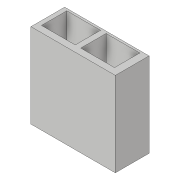
# Autodesk Inventor part: exploration1.1
Saved by Autodesk Inventor 2019 (Build 230136000, 136)
## iProperties
Created: 2020-02-18
Part Number: exploration1.1
Material: Generic
Document SubType Name: Modeling
Designer: Sandeep Shankar P
Density: 1 g/cm^3
Appearance: Default
Author: Sandeep Shankar P
Autodesk Inventor part; units mm, degrees
ref_plane "YZ Plane" through (0, 0, 0) normal (1, 0, 0) x (0, 1, 0)
ref_plane "XZ Plane" through (0, 0, 0) normal (0, 1, 0) x (-1, 0, 0)
ref_plane "XY Plane" through (0, 0, 0) normal (0, 0, 1) x (1, 0, 0)
sketch "Sketch1" plane through (0, 0, 0) normal (0, 0, 1) x (1, 0, 0)
  line L0 (-100, -49.8579) -> (100, -49.8579)
  line L1 (100, -49.8579) -> (100, 150.1421)
  line L2 (100, 150.1421) -> (-100, 150.1421)
  line L3 (-100, 150.1421) -> (-100, -49.8579)
  line L4 (-100, -49.8579) -> (100, 150.1421) construction
  line L5 (100, -49.8579) -> (-100, 150.1421) construction
  point P0 (0, 50.1421)
  dimension "d13" = 200
  dimension "d14" = 200
  dimension "d17" = 200
  constraints: 12 end point, 2 midpoint, 2 parallel, 1 horizontal, 1 perpendicular
  measures "d13" distance between parallel lines of L1 L3
  measures "d14" distance between parallel lines of L2 L0
  measures "d17" distance of L0.start L0.end
extrude "Extrusion1" add sketch "Sketch1" along normal blind 80
sketch "Sketch2" plane through (-100, 150.1421, 0) normal (0, 1, 0) x (1, 0, 0)
  line L0 (90, -65) -> (10, -65)
  line L1 (10, -65) -> (10, -5)
  line L2 (10, -5) -> (90, -5)
  line L3 (90, -5) -> (90, -65)
  line L4 (90, -65) -> (10, -5) construction
  line L5 (10, -65) -> (90, -5) construction
  line L6 (0, 0) -> (0, -80) projected
  line L7 (200, 0) -> (0, 0) projected
  point P0 (100, 0)
  point P1 (50, -35)
  dimension "d7" = 80
  dimension "d8" = 60
  dimension "d9" = 10
  dimension "d10" = 5
  constraints: 12 end point, 2 midpoint, 2 parallel, 1 horizontal, 1 perpendicular
  measures "d7" distance of L1.end L2.end
  measures "d8" distance of L0.end L1.end
  measures "d9" distance between parallel lines of L6 L1
  measures "d10" distance between parallel lines of L7 L2
extrude "Extrusion2" cut sketch "Sketch2" against normal blind 80
sketch "Sketch3" plane through (0, 0, 0) normal (0, 0, -1) x (-1, 0, 0)
  circle A0 centre (-10, 30.1421) radius 25
  line L0 (100, -49.8579) -> (-100, -49.8579) projected
  line L1 (-100, -49.8579) -> (-100, 150.1421) projected
  point P0 (0, 0)
  dimension "d19" = 50
  dimension "d20" = 80
  dimension "d21" = 90
  constraints: 1 centre point
  measures "d19" diameter of A0
  measures "d20" distance from line of L0 A0.centre
  measures "d21" distance from line of L1 A0.centre
extrude "Extrusion3" cut sketch "Sketch3" against normal blind 70
sketch "Sketch4" plane through (-100, 150.1421, 0) normal (0, 1, 0) x (1, 0, 0)
  line L0 (183.0719, -5) -> (103.0719, -5)
  line L1 (103.0719, -5) -> (103.0719, -65)
  line L2 (103.0719, -65) -> (183.0719, -65)
  line L3 (183.0719, -65) -> (183.0719, -5)
  line L4 (183.0719, -5) -> (103.0719, -65) construction
  line L5 (103.0719, -5) -> (183.0719, -65) construction
  line L6 (200, 0) -> (0, 0) projected
  point P0 (100, 0)
  point P1 (143.0719, -35)
  dimension "d24" = 80
  dimension "d25" = 60
  dimension "d26" = 5
  constraints: 12 end point, 2 midpoint, 2 parallel, 1 horizontal, 1 perpendicular
  measures "d24" distance of L2.end L1.end
  measures "d25" distance between parallel lines of L2 L0
  measures "d26" distance between parallel lines of L0 L6
extrude "Extrusion4" cut sketch "Sketch4" against normal blind 80
sketch "Sketch5" plane through (0, 0, 0) normal (0, 0, -1) x (-1, 0, 0)
  circle A0 centre (79.1012, -24.0908) radius 4.5958
  circle A1 centre (-75.3074, -24.0908) radius 4.8585
  point P0 (0, 0)
  constraints: 2 centre point
extrude "Extrusion5" cut sketch "Sketch5" against normal blind 45
body "Solid1"
